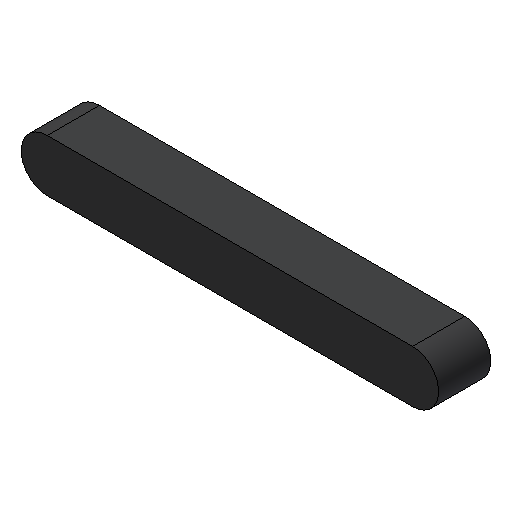
# Autodesk Inventor part: KEY
Saved by Autodesk Inventor 2022.5 (Build 265521000, 521)
## iProperties
Created: 2023-03-30
Part Number: KEY
Material: SCM435
Description: 3
Document SubType Name: Modeling
Designer: 박성규
Density: 7.84905 g/cm^3
Appearance: 일반
DETAIL: Coveryor Assembly
M/C TITLE: CJ 제일제당 협동로봇 포장시스탬 PILOT 장비
MAKER: STD
PARTS NAME: Bracket
SPECIFICATION: TA20221101-CV200000-015
DocNumber: 221118_Standard_v1
Folder: .\
VDS_Category: 엔지니어링
Detail Description: Purchased products
Title: 6x6x48L(BR)
Author: 박성규
Revision Number: A
Autodesk Inventor part; units mm, degrees
ref_plane "YZ Plane" through (0, 0, 0) normal (1, 0, 0) x (0, 1, 0)
ref_plane "XZ Plane" through (0, 0, 0) normal (0, 1, 0) x (-1, 0, 0)
ref_plane "XY Plane" through (0, 0, 0) normal (0, 0, 1) x (1, 0, 0)
sketch "스케치9" plane through (0, 0, 0) normal (0, 0, 1) x (1, 0, 0)
  line L0 (-21, 0) -> (21, 0) construction
  line L1 (-21, -3) -> (21, -3)
  line L2 (21, 3) -> (-21, 3)
  arc A0 (-21, 3) -> (-21, -3) centre (-21, 0) ccw
  arc A1 (21, -3) -> (21, 3) centre (21, 0) ccw
  point P0 (0, 0)
  point P1 (24, 0)
  point P2 (-24, 0)
  dimension "d40" = 6
  dimension "d41" = 48
  constraints: 8 end point, 6 point on circle, 4 tangent, 2 centre point, 1 horizontal, 1 midpoint, 1 parallel
  measures "d40" distance between parallel lines of L2 L1
  measures "d41" distance of point (24, 0) point (-24, 0)
extrude "돌출4" add sketch "스케치9" along normal mid plane 6
